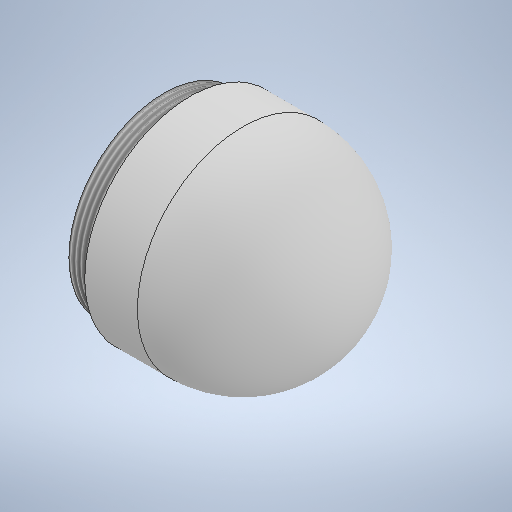
# Autodesk Inventor part: Bacteria Membrane Half 2
Saved by Autodesk Inventor 2025 (Build 290162000, 162)
## iProperties
Created: 2024-08-12
Part Number: Bacteria Membrane Half 2
Material: Generic
Document SubType Name: Modeling
Designer: kellst1
Density: 1 g/cm^3
Appearance: Default
Author: kellst1
Autodesk Inventor part; units mm, degrees
ref_plane "YZ Plane" through (0, 0, 0) normal (1, 0, 0) x (0, 1, 0)
ref_plane "XZ Plane" through (0, 0, 0) normal (0, 1, 0) x (-1, 0, 0)
ref_plane "XY Plane" through (0, 0, 0) normal (0, 0, 1) x (1, 0, 0)
sketch "Sketch1" plane through (0, 0, 0) normal (1, 0, 0) x (0, 1, 0)
  arc A0 (0, -80) -> (0, 80) centre (0, 0) ccw
  arc A1 (0, -65) -> (0, 65) centre (0, 0) ccw
  line L0 (0, 80) -> (0, 65)
  line L1 (0, -65) -> (0, -80)
  dimension "d0" = 160
  dimension "d1" = 130
  constraints: 4 end point, 4 point on circle, 2 centre point, 2 coincident, 2 vertical
  measures "d0" diameter of A0
  measures "d1" diameter of A1
revolve "Revolution1" add sketch "Sketch1" angle 180 about axis through (0, 0, 80) along (0, 0, -1)
sketch "Sketch2" plane through (0, 0, 0) normal (-1, 0, 0) x (0, 0, 1)
  circle A0 centre (0, 0) radius 80
  circle A1 centre (0, 0) radius 65
  constraints: 2 centre point, 2 coincident
extrude "Extrusion1" add sketch "Sketch2" along normal blind 40
sketch "Sketch4" plane through (-40, 0, 0) normal (-1, 0, 0) x (0, 0, 1)
  circle A0 centre (0, 0) radius 65
  circle A1 centre (0, 0) radius 72
  dimension "d8" = 144
  dimension "d9" = 130
  constraints: 2 centre point, 2 coincident
  measures "d8" diameter of A1
  measures "d9" diameter of A0
extrude "Extrusion3" add sketch "Sketch4" along normal blind 20
thread "Thread1" size "M50x4" class "6g" standard "ANSI Metric M Profile" length 20
body "Solid1"
